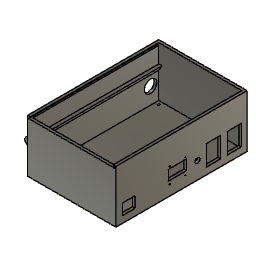
Gateway Enclosure (Autodesk Fusion 360 design; units mm, degrees)
Autodesk Fusion 360 part; units mm, degrees
box "BoxPrimitive1" add length 193 width 130 height 77.5 placed x (0, 1, 0) y (-1, 0, 0) z (0, 0, 1) at (80, 0, 0) makes body 1 in component "Box"
shell "Shell1" thickness 4 removed faces 1 at (36.6667, 64.3333, 77.5) on bodies 1 in component "Box"
sketch "Sketch2" plane through (0, 0, 0) normal (0, -1, 0) x (1, 0, 0) in component "Box"
  line L0 (-50, 77.5) -> (-50, 0)
  line L1 (-50, 0) -> (80, 0)
  line L2 (80, 0) -> (80, 77.5)
  line L3 (80, 77.5) -> (-50, 77.5)
  line L4 (76, 77.5) -> (78.2943, 74.2234)
  line L5 (76, 77.5) -> (80, 77.5) construction
  line L6 (15, 77.5) -> (15, 74.2234) construction
  line L7 (15, 74.2234) -> (78.2943, 74.2234)
  line L8 (15, 74.2234) -> (-48.2943, 74.2234)
  line L9 (-46, 77.5) -> (-48.2943, 74.2234)
  point P0 (-46, 77.5)
  point P1 (76, 77.5)
  dimension "d7" = 55
  dimension "d8" = 4
  constraint horizontal L5
  constraint coincident P1 L4.start
  constraint coincident L2.end L3.start
  constraint midpoint L3 L6.start
  constraint perpendicular L3 L6
  constraint horizontal L4.end L6.end
  constraint symmetric P1 L6 P0
  constraint symmetric L4.end L6 L8.end
  constraint symmetric L7.start L6 L8.start
  measures "d7" angle of L4 L5
  measures "d8" distance of P1 L4.end
extrude "Extrude1" cut sketch "Sketch2" against normal up to surface (189 mm away) contours L3 L4 L7 L8 L9 bodies 1 in component "Box"
sketch "Sketch1" plane through (0, 0, 0) normal (0, -1, 0) x (1, 0, 0) in component "Lid"
  line L0 (-48.2943, 74.2234) -> (-46, 77.5)
  line L1 (-46, 77.5) -> (-50, 77.5)
  line L2 (-50, 77.5) -> (-50, 0)
  line L3 (-50, 0) -> (80, 0)
  line L4 (80, 0) -> (80, 77.5)
  line L5 (80, 77.5) -> (76, 77.5)
  line L6 (76, 77.5) -> (78.2943, 74.2234)
  line L7 (78.2943, 74.2234) -> (-48.2943, 74.2234)
  line L8 (-48.2943, 74.2234) -> (-46, 77.5)
  line L9 (78.2943, 74.2234) -> (-48.2943, 74.2234)
  line L10 (-46, 77.5) -> (76, 77.5)
  line L11 (76, 77.5) -> (78.2943, 74.2234)
  line L12 (80, 77.8) -> (75.4237, 77.8)
  line L13 (75.4237, 77.8) -> (77.718, 74.5234)
  line L14 (77.718, 74.5234) -> (-47.718, 74.5234)
  line L15 (-47.718, 74.5234) -> (-45.4237, 77.8)
  line L16 (-45.4237, 77.8) -> (-50, 77.8)
  line L17 (-45.6338, 77.5) -> (75.6338, 77.5)
  dimension "d11" = 0.3
  constraint coincident L10 L17.start
  constraint coincident L15 L17.start
  constraint coincident L13 L17.end
  constraint coincident L10 L17.end
extrude "Extrude1'" add sketch "Sketch1" against normal up to surface (188.7 mm away) separate body contours L10 L13 L14 L15 L17 makes body 2 in component "Lid"
sketch "Sketch2 (2)" plane through (0, 0, 0) normal (0, -1, 0) x (1, 0, 0) in component "Lid"
  line L0 (-45.6338, 77.5) -> (-47.718, 74.5234)
  line L1 (-47.718, 74.5234) -> (77.718, 74.5234)
  line L2 (77.718, 74.5234) -> (75.6338, 77.5)
  line L3 (75.6338, 77.5) -> (-45.6338, 77.5)
  ellipse E0 centre (15, 77.5) end of major axis (22, 77.5) minor radius 0.6667
  line L4 (8, 77.5) -> (22, 77.5)
  line L5 (15, 76.8333) -> (15, 78.1667)
  dimension "d19" = 1.3333
  constraint midpoint L3 E0.centre
  constraint parallel L3 L4
  constraint coincident E0 L4.start
  constraint coincident E0 L4.end
  constraint coincident E0 L5.start
  constraint coincident E0 L5.end
extrude "Extrude2" cut sketch "Sketch2 (2)" along normal blind 5 from surface at -10 contours L3 E0 L4 L5 | L3 E0 L4 L5 | L3 E0 L4 L5 | L3 E0 L4 L5 bodies 2 in component "Lid"
sketch "Sketch3" plane through (80, 0, 0) normal (1, 0, 0) x (0, 1, 0) in component "Box"
  line L0 (0, 77.5) -> (0, 0)
  line L1 (0, 0) -> (193, 0)
  line L2 (193, 0) -> (193, 77.5)
  line L3 (193, 77.5) -> (0, 77.5)
  line L4 (164, 40) -> (185, 40)
  line L5 (185, 40) -> (185, 10)
  line L6 (185, 10) -> (164, 10)
  line L7 (164, 10) -> (164, 40)
  line L8 (133, 40) -> (154, 40)
  line L9 (154, 40) -> (154, 10)
  line L10 (154, 10) -> (133, 10)
  line L11 (133, 10) -> (133, 40)
  circle A0 centre (120, 25) radius 3.65
  line L12 (77, 35.0926) -> (104, 35.0926)
  line L13 (104, 35.0926) -> (104, 20.0926)
  line L14 (104, 20.0926) -> (77, 20.0926)
  line L15 (77, 20.0926) -> (77, 35.0926)
  circle A1 centre (79, 38.0926) radius 1
  circle A2 centre (79, 15.0926) radius 1
  line L16 (90.5, 41) -> (90.5, 10.3458) construction
  circle A3 centre (102, 38.0926) radius 1
  circle A4 centre (102, 15.0926) radius 1
  line L17 (10, 10) -> (28, 10)
  line L18 (28, 10) -> (28, 26)
  line L19 (28, 26) -> (10, 26)
  line L20 (10, 26) -> (10, 10)
  dimension "d29" = 7.3
  dimension "d30" = 27
  dimension "d31" = 15
  dimension "d32" = 2
  dimension "d33" = 2
  dimension "d58" = 18
  dimension "d59" = 16
  dimension "d64" = 30
  dimension "d65" = 21
  dimension "d66" = 21
  dimension "d67" = 30
  constraint horizontal L4
  constraint vertical L5
  constraint horizontal L6
  constraint vertical L7
  constraint horizontal L8
  constraint vertical L9
  constraint horizontal L10
  constraint vertical L11
  constraint horizontal L12
  constraint vertical L13
  constraint horizontal L14
  constraint vertical L15
  constraint perpendicular L14 L16
  constraint symmetric A1 L16 A3
  constraint symmetric A2 L16 A4
  constraint horizontal L17
  constraint vertical L18
  constraint horizontal L19
  constraint vertical L20
  measures "d29" diameter of A0
  measures "d30" distance of L12.start L12.end
  measures "d31" distance of L12.start L14.end
  measures "d32" diameter of A1
  measures "d33" diameter of A2
  measures "d58" distance of L17.start L17.end
  measures "d59" distance of L17.start L19.end
  measures "d64" distance of L8.end L10
  measures "d65" distance of L8.start L8.end
  measures "d66" distance of L4.start L4.end
  measures "d67" distance of L4.start L6.end
extrude "Extrude5" cut sketch "Sketch3" against normal up to surface (4 mm away) contours L17 L18 L19 L20 bodies 1 in component "Box"
extrude "Extrude2'" cut sketch "Sketch3" against normal up to surface (4 mm away) contours L4 L5 L6 L7 | L8 L9 L10 L11 | A0 | L12 L13 L14 L15 | A1 | A2 | A3 | A4 bodies 1 in component "Box"
sketch "Sketch4" plane through (-50, 0, 0) normal (-1, 0, 0) x (0, -1, 0) in component "Box"
  line L0 (-193, 77.5) -> (-193, 0)
  line L1 (-193, 0) -> (0, 0)
  line L2 (0, 0) -> (0, 77.5)
  line L3 (0, 77.5) -> (-193, 77.5)
  circle A0 centre (-177, 28) radius 9.25
  line L4 (-15, 15) -> (-25, 15)
  line L5 (-25, 15) -> (-25, 45)
  line L6 (-25, 45) -> (-15, 45)
  line L7 (-15, 45) -> (-15, 15)
  line L8 (-125, 45) -> (-115, 45)
  line L9 (-115, 45) -> (-115, 15)
  line L10 (-115, 15) -> (-125, 15)
  line L11 (-125, 15) -> (-125, 45)
  dimension "d40" = 18.5
  dimension "d115" = 10
  dimension "d116" = 30
  constraint horizontal L4
  constraint vertical L5
  constraint horizontal L6
  constraint vertical L7
  constraint horizontal L8
  constraint vertical L9
  constraint horizontal L10
  constraint vertical L11
  measures "d40" diameter of A0
  measures "d115" distance of L4.start L4.end
  measures "d116" distance of L4.start L6.end
extrude "Extrude10" add sketch "Sketch4" along normal blind 20 contours L8 L9 L10 L11 bodies 1 in component "Box"
extrude "Extrude9" add sketch "Sketch4" along normal blind 20 contours L4 L5 L6 L7 bodies 1 in component "Box"
extrude "Extrude3" cut sketch "Sketch4" against normal up to surface (4 mm away) contours A0 bodies 1 in component "Box"
sketch "Sketch5" plane through (0, 0, 4) normal (0, 0, 1) x (-1, 0, 0) in component "Box"
  line L0 (-76, -189) -> (46, -189)
  line L1 (46, -189) -> (46, -4)
  line L2 (46, -4) -> (-76, -4)
  line L3 (-76, -4) -> (-76, -189)
  circle A0 centre (40.46, -183.46) radius 1.75
  circle A1 centre (-38, -148) radius 1.75
  circle A2 centre (40, -41) radius 1.75
  circle A3 centre (-34, -92) radius 1.75
  dimension "d45" = 3.5
  dimension "d48" = 3.5
  dimension "d51" = 3.5
  dimension "d54" = 3.5
  measures "d45" diameter of A0
  measures "d48" diameter of A1
  measures "d51" diameter of A2
  measures "d54" diameter of A3
extrude "Extrude4" cut sketch "Sketch5" against normal up to surface (4 mm away) contours A0 | A1 | A2 | A3 bodies 1 in component "Box"
sketch "Sketch8" plane through (0, 193, 0) normal (0, 1, 0) x (-1, 0, 0) in component "Box"
  line L0 (-80, 77.5) -> (-80, 0)
  line L1 (-80, 0) -> (50, 0)
  line L2 (50, 0) -> (50, 77.5)
  line L3 (50, 77.5) -> (-80, 77.5)
  line L4 (-71, 50.5) -> (-76, 50.5)
  line L5 (-76, 50.5) -> (-76, 42.5)
  line L6 (-76, 42.5) -> (-71, 50.5)
  line L7 (-15, 77.5) -> (-15, 38.8075) construction
  line L8 (46, 42.5) -> (41, 50.5)
  line L9 (41, 50.5) -> (46, 50.5)
  line L10 (46, 50.5) -> (46, 42.5)
  dimension "d93" = 8
  constraint horizontal L4
  constraint vertical L5
  constraint midpoint L3 L7.start
  constraint perpendicular L3 L7
  constraint symmetric L5.end L7 L8.start
  constraint symmetric L4.start L7 L8.end
  constraint symmetric L4.end L7 L9.end
  measures "d93" distance of L5.end L4.end
extrude "Extrude8" add sketch "Sketch8" against normal up to surface (193 mm away) contours L4 L5 L6 | L8 L9 L10 bodies 1 in component "Box"
sketch "Sketch1 (2)" plane through (-46, 0, 0) normal (1, 0, 0) x (0, 1, 0) in component "Level (1)"
  line L0 (4, 50.5) -> (189, 50.5)
  line L1 (189, 50.5) -> (189, 74.2234)
  line L2 (189, 74.2234) -> (4, 74.2234)
  line L3 (4, 74.2234) -> (4, 50.5)
  line L4 (4.3, 74.2234) -> (4.3, 50.8)
  line L5 (4.3, 50.8) -> (188.7, 50.8)
  line L6 (188.7, 50.8) -> (188.7, 74.2234)
  line L7 (4.3, 54.2) -> (188.7, 54.2)
  constraint coincident L4 L7.start
  constraint coincident L6 L7.end
  constraint perpendicular L6 L7
extrude "Extrude1''" add sketch "Sketch1 (2)" along normal up to surface (121.4 mm away) from surface at 0.3 separate body contours L4 L5 L6 L7 makes body 3 in component "Level (1)"
sketch "Sketch2 (3)" plane through (0, 0, 54.2) normal (0, 0, 1) x (-1, 0, 0) in component "Level (1)"
  line L0 (-75.7, -4.3) -> (-75.7, -188.7)
  line L1 (-75.7, -188.7) -> (45.7, -188.7)
  line L2 (45.7, -188.7) -> (45.7, -4.3)
  line L3 (45.7, -4.3) -> (-75.7, -4.3)
  line L4 (15, -10) -> (15, -4.3)
  line L5 (15, -4.3) -> (-45, -4.3)
  line L6 (-45, -4.3) -> (-45, -24.3)
  line L7 (-45, -24.3) -> (15, -24.3)
  line L8 (15, -24.3) -> (15, -4.3)
  line L9 (-15, -4.3) -> (-15, -160) construction
  line L10 (25, -182.5663) -> (30, -182.5663)
  line L11 (30, -182.5663) -> (30, -167.5663)
  line L12 (30, -167.5663) -> (25, -167.5663)
  line L13 (25, -167.5663) -> (25, -182.5663)
  line L14 (25, -65) -> (30, -65)
  line L15 (30, -65) -> (30, -80)
  line L16 (30, -80) -> (25, -80)
  line L17 (25, -80) -> (25, -65)
  line L18 (-55, -182.5663) -> (-60, -182.5663)
  line L19 (-55, -167.5663) -> (-55, -182.5663)
  line L20 (-60, -182.5663) -> (-60, -167.5663)
  line L21 (-60, -167.5663) -> (-55, -167.5663)
  line L22 (-60, -65) -> (-60, -80)
  line L23 (-60, -80) -> (-55, -80)
  line L24 (-55, -80) -> (-55, -65)
  line L25 (-55, -65) -> (-60, -65)
  dimension "d101" = 60
  dimension "d102" = 20
  dimension "d104" = 5
  dimension "d105" = 15
  dimension "d106" = 5
  dimension "d107" = 15
  constraint coincident L3 L4.end
  constraint perpendicular L3 L4
  constraint horizontal L5
  constraint vertical L6
  constraint horizontal L7
  constraint vertical L8
  constraint midpoint L3 L9.start
  constraint perpendicular L5 L9
  constraint horizontal L10
  constraint vertical L11
  constraint horizontal L12
  constraint vertical L13
  constraint horizontal L14
  constraint vertical L15
  constraint horizontal L16
  constraint vertical L17
  constraint symmetric L9 L10.start L18.start
  constraint symmetric L9 L10.end L18.end
  constraint symmetric L9 L11.end L20.end
  constraint symmetric L9 L12.end L19.start
  constraint symmetric L9 L14.start L24.end
  constraint symmetric L9 L14.end L22.start
  constraint symmetric L9 L15.end L22.end
  constraint symmetric L9 L16.end L23.end
  measures "d101" distance of L4.end L5.end
  measures "d102" distance of L4.end L7.end
  measures "d104" distance of L10.start L10.end
  measures "d105" distance of L10.start L12.end
  measures "d106" distance of L14.start L14.end
  measures "d107" distance of L14.start L16.end
extrude "Extrude2''" cut sketch "Sketch2 (3)" against normal up to surface (3.4 mm away) contours L3 L4 L5 L6 L7 L8 | L10 L11 L12 L13 | L14 L15 L16 L17 | L18 L19 L20 L21 | L22 L23 L24 L25 bodies 3 in component "Level (1)"
sketch "Sketch10" plane through (5.1327, 15, -5.831) normal (0, -1, 0) x (1, 0, 0) in component "Box"
  line L0 (-55.1327, 20.831) -> (-55.1327, 50.831)
  line L1 (-55.1327, 50.831) -> (-75.1327, 50.831)
  line L2 (-75.1327, 50.831) -> (-75.1327, 20.831)
  line L3 (-75.1327, 20.831) -> (-55.1327, 20.831)
  spline S0 degree 2 poles (-55.1327, 20.831) (-82.6327, 35.831) (-55.1327, 50.831) knots 0 0 0 4.88083 4.88083 4.88083 weights 1 2.333333 1
  circle A0 centre (-63.1327, 35.831) radius 5
  dimension "d123" = 10
  constraint coincident L0.end L1.start
  constraint coincident L0.start L3.end
  measures "d123" diameter of A0
extrude "Extrude12" cut sketch "Sketch10" against normal up to surface (110 mm away) contours L1 L2 L3 S0 | A0 bodies 1 in component "Box"
extrude "Extrude11" [suppressed] in component "Box"
extrude "Extrude6" [suppressed] in component "Box"
sketch "Sketch7" plane through (0, 0, 0) normal (0, -1, 0) x (1, 0, 0) in component "Box"
  line L0 (-48.2943, 71.7234) -> (-46, 75)
  line L1 (-46, 75) -> (-50, 75)
  line L2 (-50, 75) -> (-50, 0)
  line L3 (-50, 0) -> (80, 0)
  line L4 (80, 0) -> (80, 75)
  line L5 (80, 75) -> (76, 75)
  line L6 (76, 75) -> (78.2943, 71.7234)
  line L7 (78.2943, 71.7234) -> (-48.2943, 71.7234)
  line L8 (71.52, 53.0261) -> (76.52, 53.0261)
  line L9 (76.52, 53.0261) -> (76.52, 45.0261)
  line L10 (76.52, 45.0261) -> (71.52, 53.0261)
  dimension "d86" = 8
  constraint horizontal L8
  constraint vertical L9
  measures "d86" distance of L9.end L8.end
extrude "Extrude7" [suppressed] in component "Box"
sketch "Sketch1 (3)" plane through (-46, 0, 0) normal (1, 0, 0) x (0, 1, 0) in component "Level"
  line L0 (4, 51) -> (189, 51)
  line L1 (189, 51) -> (189, 71.7234)
  line L2 (189, 71.7234) -> (4, 71.7234)
  line L3 (4, 71.7234) -> (4, 51)
component "Box" placed x (1, 0, 0) y (0, 1, 0) z (0, 0, 1) at (0, 0, 0)
component "Lid" placed x (1, 0, 0) y (0, 1, 0) z (0, 0, 1) at (0, 0, 0)
component "Level (1)" placed x (1, 0, 0) y (0, 1, 0) z (0, 0, 1) at (0, 0, 0)
equation "d1 = Length"
equation "d2 = Width"
equation "d3 = Height"
equation "d6 = Thickness"
equation "d8 = Thickness"
equation "d11 = Clearance"
equation "d12 = Clearance"
equation "Length = 193 mm"
equation "Width = 130 mm"
equation "Height = 77.5 mm"
equation "Thickness = 4 mm"
equation "Clearance = 0.3 mm"
equation "d19 = Thickness / 3"
equation "d28 = Length / 2"
equation "d64 = Switch_L"
equation "d65 = Switch_W"
equation "d66 = Switch_W"
equation "d67 = Switch_L"
equation "Switch_L = 30 mm"
equation "Switch_W = 21 mm"
equation "d96 = -Clearance"
equation "d98 = Clearance"
equation "d99 = Clearance"
